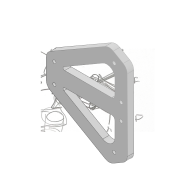
# Autodesk Inventor part: ShoulderBracket
Saved by Autodesk Inventor 2020 (Build 240168000, 168)
## iProperties
Created: 2020-04-01
Part Number: ShoulderBracket
Material: Generic
Document SubType Name: Modeling
Designer: valer
Density: 1 g/cm^3
Appearance: Default
Author: valer
Autodesk Inventor part; units mm, degrees
ref_plane "YZ Plane" through (0, 0, 0) normal (1, 0, 0) x (0, 1, 0)
ref_plane "XZ Plane" through (0, 0, 0) normal (0, 1, 0) x (-1, 0, 0)
ref_plane "XY Plane" through (0, 0, 0) normal (0, 0, 1) x (1, 0, 0)
sketch "Base" plane through (0, 0, 0) normal (0, 0, 1) x (1, 0, 0)
  line L0 (-63.5, 11.4086) -> (-63.5, -11.4086)
  line L1 (0, 31.75) -> (-14.1339, 39.9102)
  line L2 (-14.1339, -39.9102) -> (0, -31.75)
  line L3 (-63.5, 11.4086) -> (-14.1339, 39.9102)
  line L4 (-63.5, -11.4086) -> (-14.1339, -39.9102)
  line L5 (0, 31.75) -> (0, -31.75)
  line L6 (-53.8226, -5.8141) -> (-9.7028, -5.8141)
  line L7 (-9.7028, -5.8141) -> (-9.7028, -31.2866)
  line L8 (-9.7028, -31.2866) -> (-53.8226, -5.8141)
  line L9 (-63.5, 0) -> (0, 0) construction
  line L10 (-53.8226, 5.8141) -> (-9.7028, 5.8141)
  line L11 (-9.7028, 5.8141) -> (-9.7028, 31.2866)
  line L12 (-9.7028, 31.2866) -> (-53.8226, 5.8141)
  dimension "d0" = 120
  dimension "d1" = 60
  dimension "d2" = 120
  dimension "d3" = 60
  dimension "d4" = 9.7028
  dimension "d5" = 9.6837
  dimension "d6" = 9.6774
  dimension "d7" = 11.6281
  dimension "d9" = 120
  dimension "d10" = 120
  dimension "d11" = 63.5
  dimension "d12" = 63.5
  constraints: 26 end point, 3 parallel, 3 symmetric about line, 2 midpoint, 2 perpendicular, 1 coincident, 1 vertical
  measures "d0" angle of L5 L2
  measures "d1" angle of L5 L4
  measures "d2" angle of L1 L5
  measures "d3" angle of L5 L3
  measures "d4" distance between parallel lines of L5 L7
  measures "d5" distance between parallel lines of L4 L8
  measures "d6" distance from line of L0 L6.start
  measures "d7" distance between parallel lines of L6 L10
  measures "d9" angle of L1 L3
  measures "d10" angle of L2 L4
  measures "d11" distance of L1.start L2.end
  measures "d12" distance between parallel lines of L0 L5
extrude "BaseFeature" add sketch "Base" along normal blind 5.08
fillet "Fillet1" radius 6.35 8 edges at (-14.1339, 39.9102, 2.54) (0, 31.75, 2.54) (-9.7028, 31.2866, 2.54) (-14.1339, -39.9102, 2.54) (0, -31.75, 2.54) (-9.7028, -31.2866, 2.54) (-63.5, 11.4086, 2.54) (-63.5, -11.4086, 2.54)
fillet "Fillet2" radius 1.27 2 edges at (-53.8226, 5.8141, 2.54) (-53.8226, -5.8141, 2.54)
sketch "Sketch2" plane through (0, 0, 5.08) normal (0, 0, 1) x (1, 0, 0)
  circle A0 centre (-10.2851, -30.2561) radius 1.27
  circle A1 centre (-4.8514, -6.35) radius 1.27
  line L0 (-9.7028, -5.8141) -> (-9.7028, -20.2881) construction
  line L1 (0, -28.0838) -> (0, 28.0838) construction
  arc A2 (-19.2278, -25.7874) -> (-9.7028, -20.2881) centre (-16.0528, -20.2881) ccw construction
  line L2 (-10.9589, -38.0771) -> (-3.175, -33.5831) construction
  line L3 (-63.5, 7.7425) -> (-63.5, -7.7425) construction
  line L4 (-63.5, 0) -> (0, 0) construction
  line L5 (0, -28.0838) -> (0, 28.0838) construction
  arc A3 (-19.2278, -25.7874) -> (-9.7028, -20.2881) centre (-16.0528, -20.2881) ccw construction
  line L6 (-10.2851, -30.2561) -> (-7.0669, -35.8301) construction
  line L7 (-10.9589, -38.0771) -> (-3.175, -33.5831) construction
  line L8 (-17.3089, 38.0771) -> (-60.325, 13.2417) construction
  line L9 (-57.15, 15.0748) -> (-57.15, -15.0748) construction
  line L10 (-60.325, -13.2417) -> (-17.3089, -38.0771) construction
  arc A4 (-60.325, 13.2417) -> (-63.5, 7.7425) centre (-57.15, 7.7425) ccw construction
  circle A5 centre (-57.15, 7.7425) radius 1.27
  circle A6 centre (-57.15, -7.7425) radius 1.27
  circle A7 centre (-10.2851, 30.2561) radius 1.27
  circle A8 centre (-4.8514, 6.35) radius 1.27
  point P0 (-9.7028, -12.1641)
  point P1 (-12.8778, -25.7874)
  dimension "d17" = 2.54
  dimension "d18" = 4.8514
  dimension "d19" = 4.8514
  dimension "d20" = 6.4364
  dimension "d21" = 5.1664
  dimension "d22" = 6.35
  dimension "d23" = 6.35
  constraints: 6 centre point, 6 end point, 3 symmetric about line, 2 equal radius, 2 midpoint, 2 perpendicular, 2 point on circle, 2 point on line, 1 coincident, 1 vertical, 3 other
  measures "d17" diameter of A1
  measures "d18" distance from line of L1 A1.centre
  measures "d19" distance from line of L0 A1.centre
  measures "d20" distance from line of L2 L6.start
  measures "d21" distance of L6.start point (-12.878, -25.787)
  measures "d22" distance from line of A1.centre L4
  measures "d23" distance between parallel lines of L3 L9
fillet "Fillet3" radius 2.54 2 edges at (-9.7028, 5.8141, 2.54) (-9.7028, -5.8141, 2.54)
extrude "Extrusion2" cut sketch "Sketch2" against normal through all
equation "\"d19\" = d18"
body "Solid1"
